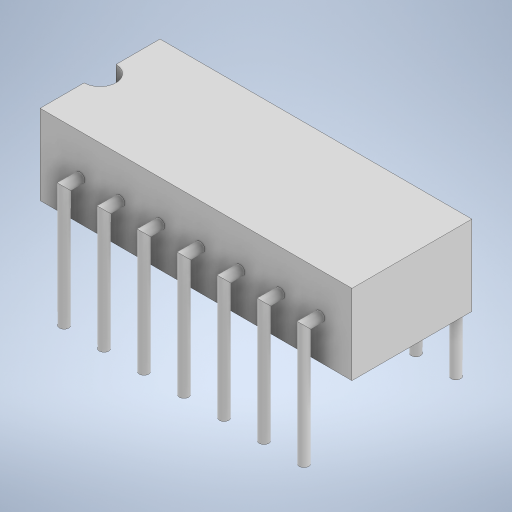
# Autodesk Inventor part: 39
Saved by Autodesk Inventor 2024 (Build 280153000, 153)
## iProperties
Created: 2023-12-01
Part Number: 39
Material: Generic
Document SubType Name: Sheet Metal
Designer: Shado
Density: 1 g/cm^3
Sheet Metal Rule: Default
Appearance: Default
Author: Shado
Autodesk Inventor part; units mm, degrees
ref_plane "YZ Plane" through (0, 0, 0) normal (1, 0, 0) x (0, 1, 0)
ref_plane "XZ Plane" through (0, 0, 0) normal (0, 1, 0) x (-1, 0, 0)
ref_plane "XY Plane" through (0, 0, 0) normal (0, 0, 1) x (1, 0, 0)
sketch "Sketch1" plane through (0, 0, 0) normal (0, 1, 0) x (-1, 0, 0)
  line L0 (0, 0) -> (0, -3.75)
  line L1 (0, -3.75) -> (19.5, -3.75)
  arc A0 (19.5, 1) -> (19.5, -1) centre (19.5, 0) ccw
  line L2 (19.5, -3.75) -> (19.5, -1)
  line L3 (0, 0) -> (0, 3.75)
  line L4 (0, 3.75) -> (19.5, 3.75)
  line L5 (19.5, 3.75) -> (19.5, 1)
  dimension "d0" = 3.75
  dimension "d1" = 19.5
  dimension "d2" = 2
  dimension "d3" = 3.75
  constraints: 12 end point, 3 perpendicular, 3 vertical, 2 point on circle, 1 centre point
  measures "d0" distance of L0.start L0.end
  measures "d1" distance of L0.end L1.end
  measures "d2" diameter of A0
  measures "d3" distance of L0.start L3.end
extrude "Extrusion1" add sketch "Sketch1" along normal blind 5
sketch "Sketch2" plane through (-19.5, 0, 3.75) normal (0, 0, 1) x (1, 0, 0)
  line L0 (0, 0) -> (0, 5) projected
  line L1 (0, 2.5) -> (19.5, 2.5)
  line L2 (19.5, 0) -> (19.5, 5) projected
  circle A0 centre (2.5, 2.5) radius 0.3
  circle A1 centre (5, 2.5) radius 0.3
  circle A2 centre (7.5, 2.5) radius 0.3
  circle A3 centre (10, 2.5) radius 0.3
  circle A4 centre (12.5, 2.5) radius 0.3
  circle A5 centre (15, 2.5) radius 0.3
  circle A6 centre (17.5, 2.5) radius 0.3
  constraints: 7 centre point, 2 midpoint, 10 other
sketch3d "3D Sketch1"
  line L0 (-17, 2.5, 3.75) -> (-17, 2.5, 4.75)
  line L1 (-17, 2.5, 4.75) -> (-17, -5, 4.75)
  dimension "d14" = 1
  dimension "d15" = 7.5
sweep "Sweep1" add profiles "Sketch2" path "3D Sketch1"
sketch "Sketch4" plane through (0, 0, -3.75) normal (0, 0, -1) x (-1, 0, 0)
  line L0 (0, 0) -> (0, 5) projected
  line L1 (19.5, 0) -> (19.5, 5) projected
  arc A0 (2.3, 2.5) -> (1.7, 2.5) centre (2, 2.5) ccw projected
  circle A1 centre (2, 2.5) radius 0.3
  circle A2 centre (4.5, 2.5) radius 0.3 projected
  circle A3 centre (4.5, 2.5) radius 0.3
  circle A4 centre (7, 2.5) radius 0.3 projected
  circle A5 centre (7, 2.5) radius 0.3
  arc A6 (9.2, 2.5) -> (9.8, 2.5) centre (9.5, 2.5) ccw projected
  circle A7 centre (9.5, 2.5) radius 0.3
  arc A8 (11.7, 2.5) -> (12.3, 2.5) centre (12, 2.5) ccw projected
  circle A9 centre (12, 2.5) radius 0.3
  circle A10 centre (14.5, 2.5) radius 0.3 projected
  circle A11 centre (14.5, 2.5) radius 0.3
  arc A12 (16.7, 2.5) -> (17.3, 2.5) centre (17, 2.5) ccw projected
  circle A13 centre (17, 2.5) radius 0.3
  constraints: 7 coincident, 4 centre point, 9 other
sketch3d "3D Sketch2"
  line L0 (-17, 2.5, -3.75) -> (-17, 2.5, -4.75)
  line L1 (-17, 2.5, -4.75) -> (-17, -5, -4.75)
sweep "Sweep2" add profiles "Sketch4" path "3D Sketch2"
equation "\"BendRadius\" = Thickness"
equation "\"BendReliefWidth\" = Thickness"
equation "\"BendReliefDepth\" = 0.5 * Thickness"
equation "\"CornerReliefSize\" = 4 * Thickness"
equation "\"MinimumRemnant\" = 2 * Thickness"
equation "\"TransitionRadius\" = BendRadius"
equation "\"JacobiRadiusSize\" = BendRadius"
equation "\"GapSize\" = Thickness"
equation "\"Thickness\" = 3.048"
body "Solid1"
